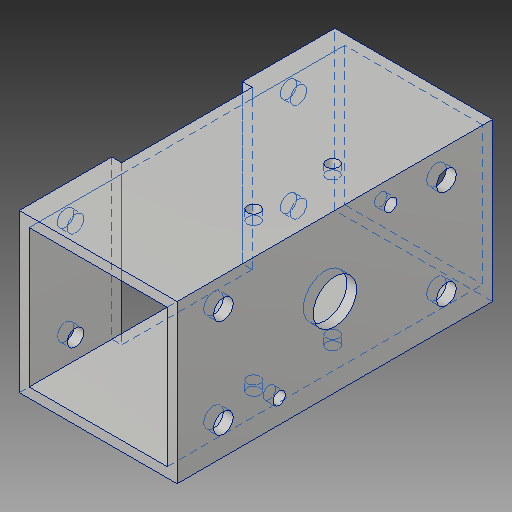
# Autodesk Inventor part: Arm 4 inch
Saved by Autodesk Inventor 2019 (Build 230136000, 136)
## iProperties
Created: 2018-09-22
Part Number: Arm 4 inch
Material: Aluminum 6061
Document SubType Name: Modeling
Designer: Adhik
Density: 2.7 g/cm^3
Appearance: Aluminum - Flat
Mass: 143.799 g
Surface Area: 361.951 cm^2
Volume: 53.2588 cm^3
Author: Adhik
Autodesk Inventor part; units mm, degrees
ref_plane "YZ Plane" through (0, 0, 0) normal (1, 0, 0) x (0, 1, 0)
ref_plane "XZ Plane" through (0, 0, 0) normal (0, 1, 0) x (-1, 0, 0)
ref_plane "XY Plane" through (0, 0, 0) normal (0, 0, 1) x (1, 0, 0)
sketch "Sketch1" plane through (0, 0, 0) normal (0, 0, 1) x (1, 0, 0)
  line L0 (-35.56, 0) -> (35.56, 0) construction
  line L1 (0, -35.56) -> (0, 35.56) construction
  line L2 (-25.4, 25.4) -> (25.4, 25.4)
  line L3 (25.4, 25.4) -> (25.4, -25.4)
  line L4 (25.4, -25.4) -> (-25.4, -25.4)
  line L5 (-25.4, -25.4) -> (-25.4, 25.4)
  line L6 (-22.225, 22.225) -> (22.225, 22.225)
  line L7 (22.225, 22.225) -> (22.225, -22.225)
  line L8 (22.225, -22.225) -> (-22.225, -22.225)
  line L9 (-22.225, -22.225) -> (-22.225, 22.225)
  point P0 (0, 0)
  point P1 (-25.4, 0)
  point P2 (0, 25.4)
  point P3 (-22.225, 0)
  point P4 (0, 22.225)
  dimension "d0" = 50.8
  dimension "d1" = 3.175
  dimension "d11" = 50.8
  dimension "d12" = 3.175
  constraints: 16 end point, 4 midpoint, 4 parallel, 4 point on line, 2 horizontal, 2 perpendicular
  measures "d0" distance of L4.end L2.start
  measures "d1" distance between parallel lines of L2 L6
  measures "d11" distance of L2.start L2.end
  measures "d12" distance between parallel lines of L5 L9
extrude "Extrusion1" add sketch "Sketch1" along normal mid plane 101.6
sketch "Sketch6" plane through (-25.4, -25.4, 50.8) normal (-1, 0, 0) x (0, 0, 1)
  line L0 (-121.92, 25.4) -> (20.32, 25.4) construction
  line L1 (-50.8, -10.16) -> (-50.8, 60.96) construction
  line L2 (-71.8058, 50.8) -> (-29.7942, 50.8)
  line L3 (-29.7942, 50.8) -> (-29.7942, 0)
  line L4 (-29.7942, 0) -> (-71.8058, 0)
  line L5 (-71.8058, 0) -> (-71.8058, 50.8)
  line L6 (-101.6, 50.8) -> (0, 50.8) construction
  point P0 (-50.8, 25.4)
  point P1 (-71.8058, 25.4)
  point P2 (-50.8, 50.8)
  dimension "d23" = 42.0116
  constraints: 8 end point, 2 midpoint, 2 parallel, 2 point on line, 1 collinear, 1 horizontal, 1 perpendicular
  measures "d23" distance of L3.end L4.end
extrude "Extrusion7" cut sketch "Sketch6" against normal blind 3.175
sketch "Sketch7" plane through (-25.4, 25.4, 50.8) normal (0, 1, 0) x (1, 0, 0)
  circle A0 centre (37.35, 38.1) radius 2.0193 projected
  circle A1 centre (37.35, 63.5) radius 2.0193 projected
  point P0 (25.4, 50.8)
extrude "Extrusion8" cut sketch "Sketch7" against normal through all
sketch "Sketch8" plane through (25.4, -25.4, 50.8) normal (1, 0, 0) x (0, 0, -1)
  line L0 (43.6, 4.4) -> (58, 4.4) construction
  line L1 (58, 4.4) -> (59.225, 3.175) construction
  line L2 (59.225, 3.175) -> (64.8, 3.175) construction
  line L3 (64.8, 9.4) -> (64.8, 3.175) construction
  arc A0 (66.8, 11.4) -> (64.8, 9.4) centre (66.8, 9.4) ccw construction
  line L4 (71.8, 11.4) -> (66.8, 11.4) construction
  line L5 (71.8, 11.4) -> (71.8, 45.4) construction
  arc A1 (71.8, 45.4) -> (70.8, 46.4) centre (50.8, 25.4) ccw construction
  line L6 (70.8, 46.4) -> (69, 46.4) construction
  line L7 (69, 46.4) -> (67.775, 47.625) construction
  line L8 (67.775, 47.625) -> (59.225, 47.625) construction
  line L9 (59.225, 47.625) -> (58, 46.4) construction
  line L10 (58, 46.4) -> (43.6, 46.4) construction
  line L11 (43.6, 46.4) -> (42.375, 47.625) construction
  line L12 (42.375, 47.625) -> (36.8, 47.625) construction
  line L13 (36.8, 41.4) -> (36.8, 47.625) construction
  arc A2 (34.8, 39.4) -> (36.8, 41.4) centre (34.8, 41.4) ccw construction
  line L14 (29.8, 39.4) -> (34.8, 39.4) construction
  line L15 (29.8, 39.4) -> (29.8, 5.4) construction
  arc A3 (29.8, 5.4) -> (30.8, 4.4) centre (50.8, 25.4) ccw construction
  line L16 (30.8, 4.4) -> (32.6, 4.4) construction
  line L17 (32.6, 4.4) -> (33.825, 3.175) construction
  line L18 (33.825, 3.175) -> (42.375, 3.175) construction
  line L19 (42.375, 3.175) -> (43.6, 4.4) construction
  circle A4 centre (50.8, 25.4) radius 14.195 construction
  circle A5 centre (32.8395, 7.4395) radius 2.0193 projected
  circle A6 centre (68.7605, 43.3605) radius 2.0193 projected
  circle A7 centre (50.8, 25.4) radius 6.985
  point P0 (50.8, 25.4)
  dimension "d28" = 13.97
  constraints: 1 centre point, 1 coincident
  measures "d28" diameter of A7
extrude "Extrusion9" cut sketch "Sketch8" against normal through all
sketch "Sketch9" plane through (-22.225, -22.225, 50.8) normal (1, 0, 0) x (0, 0, -1)
  circle A0 centre (86.7029, 6.35) radius 3.175 construction
  circle A1 centre (86.7029, 38.1) radius 3.175 construction
  circle A2 centre (14.8971, 6.35) radius 3.175 construction
  circle A3 centre (14.8971, 38.1) radius 3.175 construction
  circle A4 centre (86.7029, 6.35) radius 2.667
  circle A5 centre (14.8971, 6.35) radius 2.667
  circle A6 centre (86.7029, 38.1) radius 2.667
  circle A7 centre (14.8971, 38.1) radius 2.667
  point P0 (50.8, 22.225)
  dimension "d31" = 5.334
  constraints: 4 centre point, 4 coincident, 3 equal radius
  measures "d31" diameter of A4
extrude "Extrusion10" cut sketch "Sketch9" against normal through all
sketch "Sketch10" plane through (25.4, -25.4, 50.8) normal (1, 0, 0) x (0, 0, -1)
  circle A0 centre (14.8971, 9.525) radius 3.175 projected
  circle A1 centre (86.7029, 9.525) radius 3.175 projected
  circle A2 centre (86.7029, 41.275) radius 3.175 projected
  circle A3 centre (14.8971, 41.275) radius 3.175 projected
  point P0 (50.8, 25.4)
extrude "Extrusion11" cut sketch "Sketch10" against normal up to next
equation "\"d12\" = d1"
body "Solid1"
